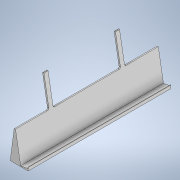
# Autodesk Inventor part: sostenedor1
Saved by Autodesk Inventor 2021 (Build 250183000, 183)
## iProperties
Created: 2021-08-01
Part Number: sostenedor1
Material: Generic
Document SubType Name: Modeling
Designer: juanc
Density: 1 g/cm^3
Appearance: Default
Author: juanc
Autodesk Inventor part; units mm, degrees
ref_plane "YZ Plane" through (0, 0, 0) normal (1, 0, 0) x (0, 1, 0)
ref_plane "XZ Plane" through (0, 0, 0) normal (0, 1, 0) x (-1, 0, 0)
ref_plane "XY Plane" through (0, 0, 0) normal (0, 0, 1) x (1, 0, 0)
sketch "Sketch1" plane through (0, 0, 0) normal (0, 0, 1) x (1, 0, 0)
  line L0 (0, 0) -> (132, 0)
  line L1 (132, 0) -> (132, 23)
  line L2 (132, 23) -> (129, 23)
  line L3 (38.7399, 220) -> (28.7399, 218.2367)
  line L4 (28.7399, 218.2367) -> (0, 0)
  line L5 (129, 23) -> (129, 15)
  line L6 (129, 15) -> (76.5186, 5.7461)
  line L7 (76.5186, 5.7461) -> (119.3723, 5.7461) construction
  line L8 (76.5186, 5.7461) -> (38.7399, 220)
  dimension "d0" = 132
  dimension "d1" = 220
  dimension "d2" = 23
  dimension "d3" = 3
  dimension "d4" = 8
  dimension "d5" = 53.291
  dimension "d6" = 10
  dimension "d7" = 90
  dimension "d8" = 10
  dimension "d9" = 10
  constraints: 18 end point, 3 perpendicular, 1 horizontal, 1 parallel
  measures "d0" distance of L0.start L0.end
  measures "d1" distance from line of L0 L3.start
  measures "d2" distance of L0.end L1.end
  measures "d3" distance of L1.end L2.end
  measures "d4" distance of L2.end L5.end
  measures "d5" distance of L5.end L6.end
  measures "d6" angle of L7 L6
  measures "d7" angle of L6 L8
  measures "d8" horizontal distance of L3.start L3.end
  measures "d9" angle of L0 L3
extrude "Extrusion1" add sketch "Sketch1" along normal blind 1050
sketch "Sketch2" plane through (28.7399, 218.2367, 1050) normal (-0.1736, 0.9848, 0) x (0.9848, 0.1736, 0)
  line L0 (10.1543, 1050) -> (10.1543, 0) construction
  line L1 (0, 277) -> (10.1543, 277)
  line L2 (10.1543, 277) -> (10.1543, 247)
  line L3 (10.1543, 247) -> (0, 247)
  line L4 (0, 247) -> (0, 277)
  line L5 (0, 1050) -> (0, 0) construction
  line L6 (0, 803) -> (10.1543, 803)
  line L7 (10.1543, 803) -> (10.1543, 773)
  line L8 (10.1543, 773) -> (0, 773)
  line L9 (0, 773) -> (0, 803)
  line L10 (10.1543, 1050) -> (0, 1050) construction
  point P0 (-66.1997, 1050)
  dimension "d12" = 30
  dimension "d13" = 30
  dimension "d14" = 247
  dimension "d15" = 247
  constraints: 16 end point, 4 parallel, 3 point on line, 2 horizontal, 2 perpendicular, 1 collinear
  measures "d12" distance between parallel lines of L3 L1
  measures "d13" distance between parallel lines of L8 L6
  measures "d14" distance between parallel lines of L10 L6
  measures "d15" distance from line of L5.end L3
extrude "Extrusion2" add sketch "Sketch2" along normal blind 220
fillet "Fillet1" radius 3 4 edges at (0.5373, 436.6577, 788) (-9.4627, 434.8944, 788) (0.5373, 436.6577, 262) (-9.4627, 434.8944, 262)
fillet "Fillet2" radius 10 4 edges at (33.7399, 219.1184, 803) (33.7399, 219.1184, 277) (33.7399, 219.1184, 773) (33.7399, 219.1184, 247)
body "Solid1"
